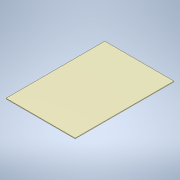
# Autodesk Inventor part: TopCoverLayer
Saved by Autodesk Inventor 2020 (Build 240168000, 168)
## iProperties
Created: 2021-01-27
Part Number: TopCoverLayer
Material: Acrylic
Document SubType Name: Modeling
Designer: abij996
Density: 1.188 g/cm^3
Appearance: Smooth - Ash
Author: abij996
Autodesk Inventor part; units mm, degrees
ref_plane "YZ Plane" through (0, 0, 0) normal (1, 0, 0) x (0, 1, 0)
ref_plane "XZ Plane" through (0, 0, 0) normal (0, 1, 0) x (-1, 0, 0)
ref_plane "XY Plane" through (0, 0, 0) normal (0, 0, 1) x (1, 0, 0)
sketch "Sketch1" plane through (0, 0, 0) normal (0, 1, 0) x (-1, 0, 0)
  line L0 (76.4554, 336.9291) -> (-273.5446, 336.9291)
  line L1 (-273.5446, 336.9291) -> (-273.5446, -163.0709)
  line L2 (-273.5446, -163.0709) -> (76.4554, -163.0709)
  line L3 (76.4554, -163.0709) -> (76.4554, 336.9291)
  point P0 (0, 0)
  dimension "d0" = 500
  dimension "d1" = 350
  constraints: 8 end point, 2 parallel, 1 horizontal, 1 perpendicular
  measures "d0" distance of L2.end L0.start
  measures "d1" distance of L1.end L2.end
extrude "Extrusion1" add sketch "Sketch1" along normal blind 3
body "Solid1"
